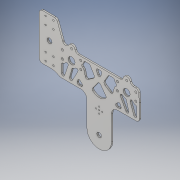
# Autodesk Inventor part: MainHolder2_2019
Saved by Autodesk Inventor 2019.4 (Build 234330000, 330)
## iProperties
Created: 2020-02-04
Part Number: MainHolder2_2019
Material: Aluminum 6061-AHC
Document SubType Name: Modeling
Designer: Paul Lefeuvre
Density: 2.7 g/cm^3
Appearance: Aluminum - Dark
Mass: 417.849 g
Surface Area: 752.79 cm^2
Volume: 154.759 cm^3
Author: Paul Lefeuvre
Autodesk Inventor part; units mm, degrees
ref_plane "YZ Plane" through (0, 0, 0) normal (1, 0, 0) x (0, 1, 0)
ref_plane "XZ Plane" through (0, 0, 0) normal (0, 1, 0) x (-1, 0, 0)
ref_plane "XY Plane" through (0, 0, 0) normal (0, 0, 1) x (1, 0, 0)
sketch "Sketch1" plane through (0, 0, 0) normal (1, 0, 0) x (0, 1, 0)
  arc A0 (-7.7083, 9.634) -> (-7.9139, 8.4066) centre (-7.1213, 8.9047) ccw
  arc A1 (-7.9139, 8.4066) -> (-7.9139, 9.4029) centre (-8.7596, 8.9047) ccw
  arc A2 (-7.6729, 9.3928) -> (-7.9139, 9.4029) centre (-7.802, 9.1932) ccw
  arc A3 (-7.9139, 9.4029) -> (-7.9139, 8.4066) centre (-7.354, 8.9047) ccw
  line L0 (-6.7058, 7.3187) -> (-6.3676, 6.5406)
  arc A4 (-6.3676, 6.5406) -> (-6.4038, 7.0491) centre (-6.5289, 6.7846) ccw
  arc A5 (-1.8791, -8.6902) -> (-2.4421, -3.7041) centre (-6.7806, -6.7188) ccw
  arc A6 (-2.4421, -3.7041) -> (-2.4421, -10.8157) centre (15.4135, -7.2599) ccw
  arc A7 (-1.8791, -8.6902) -> (-2.4421, -10.8157) centre (0.8531, -10.5512) ccw
  arc A8 (-7.7083, 9.634) -> (-7.9139, 8.4066) centre (-7.1213, 8.9047) ccw
  arc A9 (-7.7083, 9.634) -> (-7.9139, 8.4066) centre (-7.1213, 8.9047) ccw
  arc A10 (10.57, 7.2558) -> (11.0752, 7.0491) centre (10.8531, 7.2269) ccw
  arc A11 (11.0752, 7.0491) -> (10.57, 7.2558) centre (10.725, 6.9139) ccw
  arc A12 (6.3937, 6.7238) -> (6.6758, 7.2558) centre (5.9766, 7.2858) ccw
  arc A13 (6.6758, 7.2558) -> (6.2108, 6.8275) centre (6.7603, 6.6974) ccw
  line L1 (6.2108, 6.8275) -> (6.3937, 6.7238)
  line L2 (-4.7462, 4.6407) -> (-2.9659, 0.5452)
  arc A14 (-2.9659, 0.5452) -> (0.0001, -0.6323) centre (-0.8912, 1.447) ccw
  line L3 (-6.9691, 4.2944) -> (-3.8561, -1.7205)
  line L4 (-3.8561, -1.7205) -> (-3.9947, -14.1442)
  line L5 (-3.9947, -14.1442) -> (0.0001, -14.1442)
  arc A15 (-1.8791, -8.6902) -> (-2.4421, -10.8157) centre (0.8531, -10.5512) ccw
  arc A16 (-1.8791, -8.6902) -> (-2.4421, -3.7041) centre (-6.7806, -6.7188) ccw
  arc A17 (0.0001, -1.7544) -> (-1.3277, -2.0726) centre (-0.345, -3.2438) ccw
  arc A18 (-0.345, -5.4845) -> (-1.3277, -2.0726) centre (-15.2776, -7.938) ccw
  arc A19 (0.0001, -5.4655) -> (-0.345, -5.4845) centre (-0.1432, -6.0074) ccw
  arc A20 (0.0001, -12.2073) -> (-0.7359, -11.5373) centre (-1.2341, -12.8237) ccw
  arc A21 (-0.7359, -11.5373) -> (-0.2198, -9.4437) centre (-5.7065, -9.2016) ccw
  arc A22 (-0.2198, -9.4437) -> (0.0001, -9.4341) centre (-0.1502, -8.5136) ccw
  line L6 (0.0001, 13.4609) -> (0.0001, -14.9224)
  circle A23 centre (-5.7628, 5.4989) radius 1.2045
  circle A24 centre (-5.7628, 8.071) radius 1.2063
  arc A25 (-5.1733, 7.0184) -> (-5.1579, 6.5406) centre (-4.9072, 6.7878) ccw
  line L7 (0.0001, 8.0711) -> (-4.5564, 8.0711)
  arc A26 (-4.1647, 8.0711) -> (-4.6168, 7.694) centre (-4.1647, 7.6115) ccw
  circle A27 centre (-8.6319, 6.5399) radius 2
  circle A28 centre (-11.5354, 8.0725) radius 1
  circle A29 centre (-11.5337, 5.4982) radius 1.25
  arc A30 (-9.8621, 4.9631) -> (-10.568, 4.9058) centre (-10.189, 4.613) ccw
  arc A31 (-10.5696, 8.4066) -> (-9.8261, 8.1443) centre (-10.1097, 8.5253) ccw
  arc A32 (-6.6624, 3.7017) -> (-8.096, 4.6131) centre (-8.1623, 2.9254) ccw
  arc A33 (-3.8706, -3.0258) -> (-4.459, -0.5555) centre (-9.1052, -2.9674) ccw
  circle A34 centre (-1.9217, -12.8237) radius 0.4137
  arc A35 (-12.2253, 6.3955) -> (-12.2254, 7.3187) centre (-12.5811, 6.8571) ccw
  circle A36 centre (-8.724, 11.4005) radius 0.8516
  circle A37 centre (-8.724, 11.4005) radius 1.9172
  circle A38 centre (-10.4105, 13.1938) radius 0.2409
  circle A39 centre (-10.4105, 13.1938) radius 0.7717
  circle A40 centre (-6.8688, 9.634) radius 0.2412
  circle A41 centre (-6.8688, 9.634) radius 0.8395
  arc A42 (-9.3499, 8.4066) -> (-9.469, 9.634) centre (-9.8857, 8.9741) ccw
  arc A43 (-7.3048, 8.0362) -> (-6.8688, 8.7945) centre (-7.457, 8.6282) ccw
  arc A44 (-6.8688, 10.9169) -> (-6.8688, 10.4735) centre (-6.1206, 10.6952) ccw
  line L8 (-5.0063, 9.0107) -> (11.4943, 9.0107)
  circle A45 centre (11.5501, 8.0774) radius 0.3421
  circle A46 centre (11.5501, 8.0774) radius 0.935
  circle A47 centre (11.5501, 5.467) radius 0.3448
  circle A48 centre (11.5501, 5.467) radius 1.1055
  circle A49 centre (8.6229, 6.5406) radius 1.0905
  circle A50 centre (8.6229, 6.5406) radius 2.0743
  circle A51 centre (5.723, 8.0774) radius 0.3518
  circle A52 centre (5.723, 8.0774) radius 1.1343
  circle A53 centre (5.723, 5.4887) radius 0.3539
  circle A54 centre (5.723, 5.4887) radius 1.1122
  arc A55 (11.6752, 7.1508) -> (11.5501, 6.5725) centre (11.7173, 6.839) ccw
  point P0 (0, 0)
  dimension "d0" = 4
  dimension "d1" = 2
  dimension "d2" = 2.5
  constraints: 68 point on circle, 56 centre point, 18 end point
  measures "d0" diameter of A27
  measures "d1" diameter of A28
  measures "d2" diameter of A29
sketch "Sketch2" plane through (0, 0, 0) normal (0, 0, 1) x (1, 0, 0)
  line L0 (18.0589, -45.2136) -> (6.1807, -79.2835)
  arc A0 (-3.5406, -77.6375) -> (6.1807, -79.2835) centre (1.4594, -77.6375) ccw
  line L1 (-3.5406, -77.6375) -> (-3.5406, -51.5097)
  arc A1 (18.0589, -45.2136) -> (8.9949, -41.0894) centre (13.3376, -43.5676) ccw
  line L2 (57.9949, -68.102) -> (63.9949, -74.102)
  arc A2 (60.4594, -82.6375) -> (63.9949, -74.102) centre (60.4594, -77.6375) ccw
  line L3 (60.4594, -82.6375) -> (52.4594, -82.6375)
  arc A3 (47.7159, -76.0564) -> (52.4594, -82.6375) centre (52.4594, -77.6375) ccw
  line L4 (47.7159, -76.0564) -> (49.7159, -70.0564)
  arc A4 (57.9949, -68.102) -> (49.7159, -70.0564) centre (54.4594, -71.6375) ccw
  arc A5 (64.6558, -17.5783) -> (64.9131, -26.0951) centre (67.4004, -21.7577) ccw
  arc A6 (64.6558, -17.5783) -> (68.8967, -10.5547) centre (59.441, -9.6375) ccw
  arc A7 (73.8733, -6.0375) -> (68.8967, -10.5547) centre (73.8733, -11.0375) ccw
  line L5 (73.8733, -6.0375) -> (85.8733, -6.0375)
  arc A8 (90.1873, -8.5097) -> (85.8733, -6.0375) centre (85.8733, -11.0375) ccw
  line L6 (90.1873, -8.5097) -> (102.7756, -29.993)
  arc A9 (100.1649, -40.789) -> (102.7756, -29.993) centre (95.8733, -34.0375) ccw
  line L7 (100.1649, -40.789) -> (82.1233, -52.2572)
  arc A10 (74.6197, -49.3622) -> (82.1233, -52.2572) centre (79.441, -48.0375) ccw
  line L8 (79.441, -190.6375) -> (79.441, -110.6375)
  arc A11 (79.441, -110.6375) -> (59.441, -90.6375) centre (59.441, -110.6375) ccw
  line L9 (59.441, -90.6375) -> (-6.1181, -90.6375)
  line L10 (-11.5406, -89.0397) -> (-11.5406, -35.1472)
  line L11 (-11.5323, -34.8588) -> (-9.949, -7.4606)
  arc A12 (0.0343, 1.9625) -> (-9.949, -7.4606) centre (0.0343, -8.0375) ccw
  line L12 (0.0343, 1.9625) -> (238.8477, 1.9625)
  arc A13 (22.6385, -76.311) -> (31.8757, -79.9818) centre (27.4594, -77.6375) ccw
  line L13 (22.6385, -76.311) -> (30.5167, -47.6786)
  arc A14 (49.9609, -45.9119) -> (42.2035, -39.8477) centre (45.5445, -43.5676) ccw
  line L14 (49.9609, -45.9119) -> (31.8757, -79.9818)
  arc A15 (97.841, -75.8567) -> (141.041, -75.8567) centre (119.441, -55.0375) ccw
  arc A16 (97.4204, -69.4146) -> (97.841, -75.8567) centre (101.441, -72.3869) ccw
  line L15 (97.4204, -69.4146) -> (115.4204, -45.0653)
  arc A17 (123.4617, -45.0653) -> (115.4204, -45.0653) centre (119.441, -48.0375) ccw
  arc A18 (114.7987, -22.8945) -> (124.0834, -22.8945) centre (119.441, -21.0375) ccw
  line L16 (114.7987, -22.8945) -> (110.7987, -12.8945)
  arc A19 (115.441, -6.0375) -> (110.7987, -12.8945) centre (115.441, -11.0375) ccw
  line L17 (115.441, -6.0375) -> (123.441, -6.0375)
  circle A20 centre (29.441, -25.6375) radius 11.1
  circle A21 centre (59.441, -9.6375) radius 3.6
  circle A22 centre (-0.559, -9.6375) radius 3.6
  circle A23 centre (-0.559, -35.6375) radius 3.6
  circle A24 centre (59.441, -35.6375) radius 3.6
  circle A25 centre (109.441, -120.6375) radius 2.1
  circle A26 centre (119.441, -120.6375) radius 2.1
  circle A27 centre (119.441, -110.6375) radius 2.1
  circle A28 centre (119.441, -130.6375) radius 2.1
  circle A29 centre (129.441, -120.6375) radius 2.1
  circle A30 centre (29.441, -25.6375) radius 10.5
  circle A31 centre (-0.559, -9.6375) radius 3 construction
  circle A32 centre (59.441, -9.6375) radius 3 construction
  circle A33 centre (59.441, -35.6375) radius 3 construction
  circle A34 centre (-0.559, -35.6375) radius 3 construction
  arc A35 (34.1142, -44.157) -> (30.5167, -47.6786) centre (35.3376, -49.005) ccw
  arc A36 (0.8286, -46.5496) -> (-3.5406, -51.5097) centre (1.4594, -51.5097) ccw
  line L18 (60.4594, -77.6375) -> (-15.314, -77.6375) construction
  circle A37 centre (-0.559, -9.6375) radius 9.5 construction
  circle A38 centre (-0.559, -35.6375) radius 11 construction
  arc A39 (-11.5323, -34.8588) -> (-11.5406, -35.1472) centre (-6.5406, -35.1472) ccw
  line L19 (119.441, -314.199) -> (119.441, 43.2781) construction
  circle A40 centre (59.441, -35.6375) radius 11 construction
  circle A41 centre (29.441, -25.6375) radius 19.1 construction
  line L20 (70.0479, -32.7231) -> (74.6197, -49.3622)
  line L21 (144.441, -145.6375) -> (94.441, -145.6375) construction
  line L22 (94.441, -145.6375) -> (94.441, -95.6375) construction
  line L23 (94.441, -95.6375) -> (144.441, -95.6375) construction
  line L24 (144.441, -95.6375) -> (144.441, -145.6375) construction
  line L25 (144.441, -145.6375) -> (94.441, -95.6375) construction
  line L26 (94.441, -145.6375) -> (144.441, -95.6375) construction
  arc A42 (0.8286, -46.5496) -> (8.9949, -41.0894) centre (-0.559, -35.6375) ccw
  arc A43 (34.1142, -44.157) -> (42.2035, -39.8477) centre (29.441, -25.6375) ccw
  arc A44 (70.0479, -32.7231) -> (64.9131, -26.0951) centre (59.441, -35.6375) ccw
  circle A45 centre (29.441, -25.6375) radius 75 construction
  line L27 (-18.9188, -29.05) -> (-66.5438, -29.05) construction
  line L28 (-66.5438, -29.05) -> (-66.5438, 18.575) construction
  line L29 (-66.5438, 18.575) -> (-18.9188, 18.575) construction
  line L30 (-18.9188, 18.575) -> (-18.9188, -29.05) construction
  line L31 (-18.9188, -29.05) -> (-66.5438, 18.575) construction
  line L32 (-66.5438, -29.05) -> (-18.9188, 18.575) construction
  circle A46 centre (-42.7313, -5.2375) radius 8
  circle A47 centre (-42.7313, -5.2375) radius 32 construction
  circle A48 centre (-42.7313, -5.2375) radius 34 construction
  line L33 (66.6134, -39.2375) -> (-45.8121, -39.2375) construction
  line L34 (-0.0862, 15.1221) -> (-17.1468, 61.9957)
  line L35 (-26.5438, 68.5755) -> (-66.5438, 68.5755)
  line L36 (-76.5438, 58.5755) -> (-76.5438, -71.0505)
  line L37 (-66.5438, -81.0505) -> (-38.6532, -81.0505)
  arc A49 (-66.5438, 68.5755) -> (-76.5438, 58.5755) centre (-66.5438, 58.5755) ccw
  arc A50 (-76.5438, -71.0505) -> (-66.5438, -81.0505) centre (-66.5438, -71.0505) ccw
  arc A51 (-17.1468, 61.9957) -> (-26.5438, 68.5755) centre (-26.5438, 58.5755) ccw
  arc A52 (-0.0862, 15.1221) -> (18.7076, 1.9625) centre (18.7076, 21.9625) ccw
  arc A53 (79.441, -190.6375) -> (79.441, -190.6375) centre (96.5576, -190.6375) ccw
  line L38 (109.441, -120.6375) -> (129.441, -120.6375) construction
  line L39 (220.8232, -45.2136) -> (232.7014, -79.2835)
  arc A54 (232.7014, -79.2835) -> (242.4227, -77.6375) centre (237.4227, -77.6375) ccw
  line L40 (242.4227, -77.6375) -> (242.4227, -51.5097)
  arc A55 (229.8872, -41.0894) -> (220.8232, -45.2136) centre (225.5445, -43.5676) ccw
  line L41 (180.8872, -68.102) -> (174.8872, -74.102)
  arc A56 (174.8872, -74.102) -> (178.4227, -82.6375) centre (178.4227, -77.6375) ccw
  line L42 (178.4227, -82.6375) -> (186.4227, -82.6375)
  arc A57 (186.4227, -82.6375) -> (191.1661, -76.0564) centre (186.4227, -77.6375) ccw
  line L43 (191.1661, -76.0564) -> (189.1661, -70.0564)
  arc A58 (189.1661, -70.0564) -> (180.8872, -68.102) centre (184.4227, -71.6375) ccw
  arc A59 (173.969, -26.0951) -> (174.2263, -17.5783) centre (171.4817, -21.7577) ccw
  arc A60 (169.9854, -10.5547) -> (174.2263, -17.5783) centre (179.441, -9.6375) ccw
  arc A61 (169.9854, -10.5547) -> (165.0088, -6.0375) centre (165.0088, -11.0375) ccw
  line L44 (165.0088, -6.0375) -> (153.0088, -6.0375)
  arc A62 (153.0088, -6.0375) -> (148.6948, -8.5097) centre (153.0088, -11.0375) ccw
  line L45 (148.6948, -8.5097) -> (136.1065, -29.993)
  arc A63 (136.1065, -29.993) -> (138.7172, -40.789) centre (143.0088, -34.0375) ccw
  line L46 (138.7172, -40.789) -> (156.7588, -52.2572)
  arc A64 (156.7588, -52.2572) -> (164.2624, -49.3622) centre (159.441, -48.0375) ccw
  line L47 (159.441, -190.6375) -> (159.441, -110.6375)
  arc A65 (179.441, -90.6375) -> (159.441, -110.6375) centre (179.441, -110.6375) ccw
  line L48 (250.4144, -34.8588) -> (248.8311, -7.4606)
  arc A66 (248.8311, -7.4606) -> (238.8477, 1.9625) centre (238.8477, -8.0375) ccw
  arc A67 (207.0064, -79.9818) -> (216.2436, -76.311) centre (211.4227, -77.6375) ccw
  line L49 (216.2436, -76.311) -> (208.3654, -47.6786)
  arc A68 (196.6785, -39.8477) -> (188.9212, -45.9119) centre (193.3376, -43.5676) ccw
  line L50 (188.9212, -45.9119) -> (207.0064, -79.9818)
  arc A69 (141.041, -75.8567) -> (141.4617, -69.4146) centre (137.441, -72.3869) ccw
  line L51 (141.4617, -69.4146) -> (123.4617, -45.0653)
  circle A70 centre (209.441, -25.6375) radius 11.1
  circle A71 centre (179.441, -9.6375) radius 3.6
  circle A72 centre (239.441, -9.6375) radius 3.6
  circle A73 centre (239.441, -35.6375) radius 3.6
  circle A74 centre (179.441, -35.6375) radius 3.6
  arc A75 (208.3654, -47.6786) -> (204.7679, -44.157) centre (203.5445, -49.005) ccw
  arc A76 (242.4227, -51.5097) -> (238.0534, -46.5496) centre (237.4227, -51.5097) ccw
  arc A77 (250.4227, -35.1472) -> (250.4144, -34.8588) centre (245.4227, -35.1472) ccw
  line L52 (168.8341, -32.7231) -> (164.2624, -49.3622)
  arc A78 (229.8872, -41.0894) -> (238.0534, -46.5496) centre (239.441, -35.6375) ccw
  arc A79 (196.6785, -39.8477) -> (204.7679, -44.157) centre (209.441, -25.6375) ccw
  arc A80 (173.969, -26.0951) -> (168.8341, -32.7231) centre (179.441, -35.6375) ccw
  line L53 (124.0834, -22.8945) -> (128.0834, -12.8945)
  arc A81 (128.0834, -12.8945) -> (123.441, -6.0375) centre (123.441, -11.0375) ccw
  circle A82 centre (29.441, -25.6375) radius 20.6 construction
  circle A83 centre (29.441, 8.3625) radius 3.6
  line L54 (29.441, -25.6375) -> (29.441, 8.3625) construction
  arc A84 (40.8788, 10.2958) -> (18.9018, 13.2085) centre (29.441, 8.3625) ccw
  arc A85 (40.8788, 10.2958) -> (50.7389, 1.9625) centre (50.7389, 11.9625) ccw
  line L55 (209.441, -25.6375) -> (209.441, 8.3625) construction
  circle A86 centre (209.441, 8.3625) radius 3.6
  arc A87 (220.8788, 10.2958) -> (198.0033, 10.2958) centre (209.441, 8.3625) ccw
  arc A88 (188.1432, 1.9625) -> (198.0033, 10.2958) centre (188.1432, 11.9625) ccw
  arc A89 (220.8788, 10.2958) -> (230.7389, 1.9625) centre (230.7389, 11.9625) ccw
  circle A90 centre (119.441, -190.6375) radius 7.5
  circle A91 centre (-55.4313, -43.6505) radius 2.6
  circle A92 centre (-30.0313, -43.6505) radius 2.6
  circle A93 centre (-30.0313, -69.0505) radius 2.6
  circle A94 centre (-55.4313, -69.0505) radius 2.6
  line L56 (-30.0313, -69.0505) -> (-55.4313, -69.0505) construction
  line L57 (-55.4313, -69.0505) -> (-55.4313, -43.6505) construction
  line L58 (-55.4313, -43.6505) -> (-30.0313, -43.6505) construction
  line L59 (-30.0313, -43.6505) -> (-30.0313, -69.0505) construction
  line L60 (-30.0313, -69.0505) -> (-55.4313, -43.6505) construction
  line L61 (-55.4313, -69.0505) -> (-30.0313, -43.6505) construction
  circle A95 centre (-55.4313, 58.5755) radius 2.6
  circle A96 centre (-30.0313, 58.5755) radius 2.6
  circle A97 centre (-30.0313, 33.1755) radius 2.6
  circle A98 centre (-55.4313, 33.1755) radius 2.6
  line L62 (-30.0313, 33.1755) -> (-55.4313, 33.1755) construction
  line L63 (-55.4313, 33.1755) -> (-55.4313, 58.5755) construction
  line L64 (-55.4313, 58.5755) -> (-30.0313, 58.5755) construction
  line L65 (-30.0313, 58.5755) -> (-30.0313, 33.1755) construction
  line L66 (-30.0313, 33.1755) -> (-55.4313, 58.5755) construction
  line L67 (-55.4313, 33.1755) -> (-30.0313, 58.5755) construction
  line L68 (-42.7313, 45.8755) -> (-42.7313, -56.3505) construction
  arc A99 (-11.5406, -89.0397) -> (-6.1181, -90.6375) centre (-6.1181, -80.6375) ccw
  arc A100 (-11.5406, -89.0397) -> (-38.6532, -81.0505) centre (-38.6532, -131.0505) ccw
  line L69 (250.4227, -35.1472) -> (250.4227, -80.6375)
  line L70 (240.4227, -90.6375) -> (179.441, -90.6375)
  arc A101 (240.4227, -90.6375) -> (250.4227, -80.6375) centre (240.4227, -80.6375) ccw
  arc A102 (79.441, -190.6375) -> (159.441, -190.6375) centre (119.441, -190.6375) ccw
  arc A103 (0.9248, 12.8098) -> (18.9018, 13.2085) centre (9.8162, 17.3862) ccw
  point P0 (0, 0)
  point P1 (-3.5406, -44.9447)
  point P2 (-11.5406, -35.0029)
  point P3 (31.303, -44.821)
  point P4 (214.556, 1.9625)
  point P5 (119.441, -120.6375)
  point P6 (119.441, -120.6375)
  point P7 (-42.7313, -56.3505)
  point P8 (-42.7313, 45.8755)
  dimension "d115" = 150
  dimension "d3" = 0.6
  dimension "d4" = 0.6
  dimension "d5" = 0.6
  dimension "d6" = 0.6
  dimension "d7" = 0.6
  dimension "d14" = 8
  dimension "d15" = 5
  dimension "d16" = 5
  dimension "d17" = 5
  dimension "d19" = 5
  dimension "d22" = 5
  dimension "d23" = 5
  dimension "d26" = 5
  dimension "d27" = 5
  dimension "d28" = 5
  dimension "d30" = 8
  dimension "d32" = 19
  dimension "d33" = 22
  dimension "d34" = 5
  dimension "d35" = 9.5
  dimension "d38" = 5
  dimension "d39" = 5
  dimension "d40" = 5
  dimension "d41" = 8
  dimension "d42" = 5
  dimension "d44" = 8
  dimension "d46" = 10
  dimension "d47" = 11.6
  dimension "d48" = 5
  dimension "d49" = 5
  dimension "d51" = 8
  dimension "d53" = 55
  dimension "d54" = 26
  dimension "d55" = 22
  dimension "d56" = 8
  dimension "d57" = 6
  dimension "d58" = 25
  dimension "d59" = 2
  dimension "d60" = 38.2
  dimension "d61" = 22
  dimension "d62" = 36
  dimension "d63" = 12
  dimension "d64" = 22
  dimension "d65" = 50
  dimension "d66" = 40
  dimension "d67" = 5
  dimension "d68" = 5
  dimension "d69" = 30
  dimension "d71" = 18
  dimension "d73" = 40
  dimension "d75" = 20
  dimension "d77" = 50
  dimension "d78" = 50
  dimension "d89" = 7
  dimension "d116" = 47.625
  dimension "d117" = 47.625
  dimension "d118" = 16
  dimension "d119" = 64
  dimension "d120" = 2
  dimension "d128" = 10
  dimension "d131" = 10
  dimension "d133" = 10
  dimension "d134" = 20
  dimension "d135" = 90
  constraints: 142 end point, 136 point on circle, 103 centre point, 72 tangent, 71 symmetric about line, 21 coincident, 16 point on line, 15 midpoint, 12 horizontal, 8 parallel, 7 perpendicular, 7 vertical, 4 equal radius, 3 line through centre, 32 other
  measures "d3" radial gap between concentric circles of A20 A30
  measures "d4" radial gap between concentric circles of A22 A31
  measures "d5" radial gap between concentric circles of A21 A32
  measures "d6" radial gap between concentric circles of A24 A33
  measures "d7" radial gap between concentric circles of A23 A34
  measures "d14" distance between parallel lines of L9 L3
  measures "d15" radius of A35
  measures "d16" radius of A36
  measures "d17" radius of A14
  measures "d19" radius of A13
  measures "d22" radius of A0
  measures "d23" radius of A1
  measures "d26" radius of A4
  measures "d27" radius of A3
  measures "d28" radius of A2
  measures "d30" distance between parallel lines of L10 L1
  measures "d32" diameter of A37
  measures "d33" diameter of A38
  measures "d34" radius of A39
  measures "d35" radius of A6
  measures "d38" radius of A5
  measures "d39" radius of A7
  measures "d40" radius of A8
  measures "d41" radius of A9
  measures "d42" radius of A10
  measures "d44" distance between parallel lines of L12 L5
  measures "d46" radius of A12
  measures "d47" distance from line of A22.centre L12
  measures "d48" radius of A19
  measures "d49" radius of A18
  measures "d51" distance of L17.end L17.start
  measures "d53" distance from line of L9 A23.centre
  measures "d54" distance of A13.centre A0.centre
  measures "d55" diameter of A40
  measures "d56" distance of L18.start A3.centre
  measures "d57" distance from line of L18 A4.centre
  measures "d58" distance of A13.centre A3.centre
  measures "d59" horizontal distance of A4.centre A3.centre
  measures "d60" diameter of A41
  measures "d61" horizontal distance of A1.centre A35.centre
  measures "d62" distance from line of L12 A9.centre
  measures "d63" distance of L5.start L5.end
  measures "d64" horizontal distance of A7.centre A9.centre
  measures "d65" distance from line of L12 A10.centre
  measures "d66" distance from line of L19 A10.centre
  measures "d67" radius of A17
  measures "d68" radius of A16
  measures "d69" radius of A15
  measures "d71" distance from line of L19 A16.centre
  measures "d73" distance between parallel lines of L8 L19
  measures "d75" radius of A11
  measures "d77" distance of L22.end L23.end
  measures "d78" distance of L21.end L22.end
  measures "d89" distance of A15.centre A17.centre
  measures "d116" distance of L28.end L29.end
  measures "d117" distance of L27.end L28.end
  measures "d118" diameter of A46
  measures "d119" diameter of A47
  measures "d120" radial gap between concentric circles of A47 A48
  measures "d128" distance between parallel lines of L36 L28
  measures "d131" radius of A49
  measures "d133" radius of A51
  measures "d134" radius of A52
  measures "d135" distance from line of L19 A20.centre
extrude "Extrusion3" add sketch "Sketch2" along normal blind 5 contours A53 A90 | L8 A11 L9 A99 L10 A39 L11 A12 L12 A66 L48 A77 L69 A101 L70 A65 L47 A102 | A100 L37 A50 L36 A49 L35 A51 L34 A52 L12 A12 L11 A39 L10 | A52 A103 A84 A85 L12 | L12 A88 A87 A89 picked at (90.4568, -192.2922)
body "Solid3"
